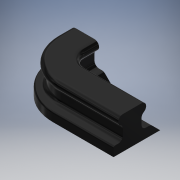
# Autodesk Inventor part: Rail Corner 2
Saved by Autodesk Inventor 2019 (Build 230136000, 136)
## iProperties
Created: 2020-12-25
Part Number: Rail Corner 2
Material: Acetal Resin, Black
Document SubType Name: Modeling
Designer: John
Density: 1.425 g/cm^3
Appearance: Smooth - Black
Author: John
Autodesk Inventor part; units mm, degrees
ref_plane "YZ Plane" through (0, 0, 0) normal (1, 0, 0) x (0, 1, 0)
ref_plane "XZ Plane" through (0, 0, 0) normal (0, 1, 0) x (-1, 0, 0)
ref_plane "XY Plane" through (0, 0, 0) normal (0, 0, 1) x (1, 0, 0)
sketch "Sketch1" plane through (0, 0, 0) normal (1, 0, 0) x (0, 1, 0)
  line L0 (-3.175, -15.8752) -> (-3.175, 15.8752)
  line L1 (-3.175, 15.8752) -> (1.9596, -9.7981) construction
  line L2 (3.175, 15.8752) -> (-3.175, -15.8752) construction
  arc A0 (18.3756, 12.7) -> (12.0256, 12.7001) centre (15.2006, 12.7) ccw
  arc A1 (12.0256, -12.7001) -> (18.3756, -12.7) centre (15.2006, -12.7) ccw
  line L3 (8.8506, 9.5252) -> (6.35, 9.5252)
  line L4 (8.8506, -9.5252) -> (5.1346, -9.5252)
  line L5 (15.2006, 12.7) -> (15.2006, -12.7) construction
  line L6 (3.175, 14.6052) -> (3.175, 12.7002)
  arc A2 (8.8506, 9.5252) -> (12.0256, 12.7001) centre (8.8506, 12.7002) ccw
  arc A3 (12.0256, -12.7001) -> (8.8506, -9.5252) centre (8.8506, -12.7002) ccw
  arc A4 (3.175, 12.7002) -> (6.35, 9.5252) centre (6.35, 12.7002) ccw
  arc A5 (5.1346, -9.5252) -> (1.9937, -12.2364) centre (5.1346, -12.7002) ccw
  line L7 (-3.175, -15.8752) -> (-3.175, -22.2252)
  line L8 (1.905, 15.8752) -> (-3.175, 15.8752)
  arc A6 (3.175, 14.6052) -> (1.905, 15.8752) centre (1.905, 14.6052) ccw
  line L9 (18.3756, 12.7) -> (18.3756, -12.7)
  line L10 (1.6475, -13.2791) -> (-3.175, -22.2252)
  arc A7 (1.6475, -13.2791) -> (1.9937, -12.2364) centre (-1.1473, -11.7726) ccw
  line L11 (-3.175, -22.2252) -> (20.4919, -22.2252)
  point P0 (0, 0)
  point P1 (15.2367, 9.5252)
  point P2 (15.2367, -9.5252)
  point P3 (1.9596, -12.7002)
  dimension "d5" = 6.35
  dimension "d8" = 3.175
  dimension "d9" = 6.35
  dimension "d11" = 6.35
  dimension "d12" = 6.35
  dimension "d13" = 1.27
  dimension "d30" = 25.4
  dimension "d31" = 3.175
  constraints: 24 end point, 19 point on circle, 13 tangent, 8 centre point, 6 point on line, 4 equal radius, 2 parallel, 2 perpendicular, 2 vertical, 1 horizontal, 1 midpoint
  measures "d5" diameter of A1
  measures "d8" radius of A2
  measures "d9" distance of L0.start L7.end
  measures "d11" distance between parallel lines of L3 L8
  measures "d12" distance from line of L0.start L4
  measures "d13" radius of A6
  measures "d30" distance of L5.start L5.end
  measures "d31" radius of A7
revolve "Revolution1" add sketch "Sketch1" angle 90 about axis through (0, -3.175, -22.2252) along (0, -1, 0)
extrude "Extrusion2" add sketch "Sketch1" along normal blind 41.275
sketch "Sketch2" plane through (-9.5252, 18.3756, -22.2252) normal (0, 0, -1) x (-1, 0, 0)
  line L0 (-9.5252, -21.5506) -> (28.5752, -21.5506) projected
  line L1 (28.5752, -21.5506) -> (28.5752, -16.4706) projected
  arc A0 (28.5752, -16.4706) -> (27.3052, -15.2006) centre (27.3052, -16.4706) ccw projected
  line L2 (27.3052, -15.2006) -> (25.4002, -15.2006) projected
  arc A1 (22.2252, -12.0256) -> (25.4002, -15.2006) centre (25.4002, -12.0256) ccw projected
  line L3 (22.2252, -12.0256) -> (22.2252, -9.525) projected
  arc A2 (25.4001, -6.35) -> (22.2252, -9.525) centre (25.4002, -9.525) ccw projected
  arc A3 (25.4001, -6.35) -> (25.4, 0) centre (25.4, -3.175) ccw projected
  line L4 (25.4, 0) -> (0, 0) projected
  arc A4 (0, 0) -> (-0.0001, -6.35) centre (0, -3.175) ccw projected
  arc A5 (3.1748, -9.525) -> (-0.0001, -6.35) centre (-0.0002, -9.525) ccw projected
  line L5 (3.1748, -9.525) -> (3.1748, -13.241) projected
  arc A6 (0.4636, -16.382) -> (3.1748, -13.241) centre (-0.0002, -13.241) ccw projected
  arc A7 (0.4636, -16.382) -> (-0.5791, -16.7281) centre (0.9274, -19.5229) ccw projected
  line L6 (-0.5791, -16.7281) -> (-9.5252, -21.5506) projected
  point P0 (-9.5252, -18.3756)
extrude "Extrusion3" add sketch "Sketch2" along normal blind 9.2075
sketch "Sketch5" plane through (41.275, 0, 0) normal (1, 0, 0) x (0, 0, -1)
  circle A0 centre (0, 7.5946) radius 2.2225
  line L0 (-15.8752, -3.175) -> (22.2252, -3.175) projected
  point P0 (0, 0)
  dimension "d26" = 4.445
  dimension "d27" = 10.7696
  constraints: 1 centre point
  measures "d26" diameter of A0
  measures "d27" distance from line of L0 A0.centre
extrude "Extrusion4" cut sketch "Sketch5" against normal blind 12.7
sketch "Sketch6" plane through (-9.5252, 18.3756, -31.4327) normal (0, 0, -1) x (-1, 0, 0)
  line L0 (3.1748, -9.525) -> (3.1748, -13.241) projected
  line L1 (3.1748, -10.781) -> (22.2252, -10.781) construction
  line L2 (22.2252, -12.0256) -> (22.2252, -9.525) projected
  circle A0 centre (12.7, -10.781) radius 2.2225
  line L3 (-9.5252, -21.5506) -> (28.5752, -21.5506) projected
  point P0 (-9.5252, -18.3756)
  dimension "d32" = 4.445
  dimension "d33" = 10.7696
  constraints: 2 end point, 2 point on line, 1 centre point, 1 horizontal, 1 midpoint
  measures "d32" diameter of A0
  measures "d33" distance between parallel lines of L3 L1
extrude "Extrusion5" cut sketch "Sketch6" against normal blind 12.7
sketch "Sketch7" plane through (0, -3.175, 15.8752) normal (0, -1, 0) x (1, 0, 0)
  line L0 (28.575, -13.6527) -> (28.575, -18.0977) projected
  line L1 (41.275, -13.6527) -> (41.275, -18.0977) projected
  line L2 (-20.0027, -34.6079) -> (-24.4477, -34.6079) projected
  line L3 (-20.0027, -47.3079) -> (-24.4477, -47.3079) projected
  line L4 (25.4, -22.2252) -> (31.75, -22.2252)
  line L5 (31.75, -22.2252) -> (31.75, -9.5252)
  line L6 (31.75, -9.5252) -> (25.4, -9.5252)
  line L7 (25.4, -9.5252) -> (25.4, -22.2252)
  line L8 (28.575, -13.6527) -> (28.575, -18.0977) projected
  line L9 (25.4, -22.2252) -> (31.75, -9.5252) construction
  line L10 (31.75, -22.2252) -> (25.4, -9.5252) construction
  line L11 (-28.5752, -31.4329) -> (-15.8752, -31.4329)
  line L12 (-15.8752, -31.4329) -> (-15.8752, -37.7829)
  line L13 (-15.8752, -37.7829) -> (-28.5752, -37.7829)
  line L14 (-28.5752, -37.7829) -> (-28.5752, -31.4329)
  line L15 (-20.0027, -34.6079) -> (-24.4477, -34.6079) projected
  line L16 (-28.5752, -31.4329) -> (-15.8752, -37.7829) construction
  line L17 (-15.8752, -31.4329) -> (-28.5752, -37.7829) construction
  point P0 (0, -15.8752)
  point P1 (28.575, -15.8752)
  point P2 (-22.2252, -34.6079)
  dimension "d36" = 12.7
  dimension "d37" = 6.35
  constraints: 24 end point, 6 midpoint, 4 parallel, 4 perpendicular, 2 horizontal
  measures "d36" distance of L6.end L4.start
  measures "d37" distance of L4.start L4.end
extrude "Extrusion6" cut sketch "Sketch7" against normal blind 17.145
fillet "Fillet1" radius 6.35 4 edges at (28.575, 13.97, -6.35) (28.575, 13.97, 6.35) (-15.8752, 13.97, -18.7327) (-28.5752, 13.97, -18.7327)
body "Solid2"
